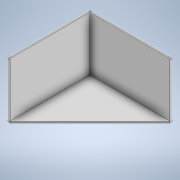
# Autodesk Inventor part: Table Corner
Saved by Autodesk Inventor 2021 (Build 250183000, 183)
## iProperties
Created: 2021-03-13
Part Number: Table Corner
Material: Generic
Document SubType Name: Modeling
Designer: dech3
Density: 1 g/cm^3
Appearance: Default
Author: dech3
Autodesk Inventor part; units mm, degrees
ref_plane "YZ Plane" through (0, 0, 0) normal (1, 0, 0) x (0, 1, 0)
ref_plane "XZ Plane" through (0, 0, 0) normal (0, 1, 0) x (-1, 0, 0)
ref_plane "XY Plane" through (0, 0, 0) normal (0, 0, 1) x (1, 0, 0)
sketch "Sketch1" plane through (0, 0, 0) normal (0, 1, 0) x (-1, 0, 0)
  line L0 (15, -12.52) -> (-25, -12.52)
  line L1 (15, 27.48) -> (15, -12.52)
  line L2 (15, 27.48) -> (-25, -12.52)
  point P0 (0, 0)
  point P1 (-25, -12.52)
  dimension "d0" = 40
  dimension "d2" = 15
  dimension "d3" = 45
  dimension "d6" = 40
  constraints: 6 end point, 3 coincident, 1 horizontal, 1 vertical
  measures "d0" distance of L0.start L1.start
  measures "d2" distance from line of point (0, 0) L1
  measures "d3" angle of L0 L2
  measures "d6" distance of L0.start L0.end
extrude "Extrusion1" add sketch "Sketch1" along normal blind 26.5
sketch "Sketch2" plane through (0, 26.5, 0) normal (0, 1, 0) x (1, 0, 0)
  line L0 (-13.5, -25.98) -> (-13.5, 11.02)
  line L1 (-13.5, 11.02) -> (23.5, 11.02)
  line L2 (23.5, 11.02) -> (-13.5, -25.98)
  line L3 (-15, -27.48) -> (25, 12.52) projected
  line L4 (25, 12.52) -> (-15, 12.52) projected
  line L5 (-15, 12.52) -> (-15, -27.48) projected
  point P0 (0, 0)
  point P1 (23.5, 11.02)
  point P2 (-13.5, 11.02)
  dimension "d8" = 0
  dimension "d9" = 1.5
  dimension "d10" = 1.5
  constraints: 6 coincident, 6 end point, 1 collinear
  measures "d8" distance between parallel lines of L3 L2
  measures "d9" distance between parallel lines of L4 L1
  measures "d10" distance between parallel lines of L5 L0
extrude "Extrusion2" cut sketch "Sketch2" against normal blind 25 contours L0 L1 L2
fillet "Fillet1" radius 1 7 edges at (-15, 26.5, 7.48) (-15, 13.25, 27.48) (5, 26.5, -12.52) (-15, 13.25, -12.52) (25, 13.25, -12.52) (5, 0, -12.52) (-15, 0, 7.48)
fillet "Fillet2" radius 1 5 edges at (23.5097, 0, -11.1373) (23.2929, 0.2929, -12.2271) (-13.6173, 0, 25.9897) (-14.7071, 0.2929, 25.7729) (5, 0, 7.48)
fillet "Fillet3" radius 0.5 4 edges at (23.5517, 26.5, -11.2611) (23.2929, 26.2071, -12.2271) (-14.7071, 26.2071, 25.7729) (-13.7412, 26.5, 26.0318)
equation "\"d6\" = d0"
body "Solid1"
